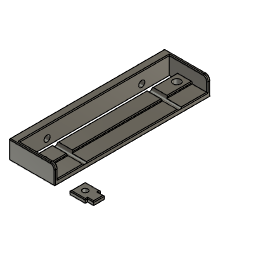
PS_LRS150-LM200_1515Mount (Autodesk Fusion 360 design; units mm, degrees)
Autodesk Fusion 360 part; units mm, degrees
sketch "Sketch1" plane through (0, 0, 0) normal (0, 0, 1) x (1, 0, 0)
  line L0 (0, 0) -> (5, 0)
  line L1 (5, 0) -> (5, 102)
  line L2 (5, 102) -> (0, 102)
  line L3 (0, 102) -> (0, 0)
  line L4 (5, 0) -> (5, 2)
  line L5 (5, 2) -> (5, 0)
  line L6 (5, 100) -> (5, 102)
  line L7 (0, 0) -> (30, 0)
  line L8 (30, 0) -> (30, 2)
  line L9 (30, 2) -> (0, 2)
  line L10 (0, 2) -> (0, 0)
  line L11 (0, 102) -> (30, 102)
  line L12 (30, 102) -> (30, 100)
  line L13 (30, 100) -> (0, 100)
  line L14 (0, 100) -> (0, 102)
  line L15 (0, 0) -> (30, 0)
  line L16 (30, 0) -> (30, 102)
  line L17 (30, 102) -> (0, 102)
  line L18 (0, 102) -> (0, 0)
  line L19 (5, 2) -> (10, 2)
  line L20 (10, 2) -> (20, 2)
  line L21 (20, 2) -> (20, 100)
  line L22 (20, 100) -> (10, 100)
  line L23 (10, 100) -> (10, 2)
  circle A0 centre (15, 7) radius 2.5
  circle A1 centre (15, 95) radius 2.5
  line L24 (40, 0) -> (54, 0)
  line L25 (54, 0) -> (54, 10)
  line L26 (54, 10) -> (40, 10)
  line L27 (40, 10) -> (40, 0)
  circle A2 centre (45, 5) radius 1.75
  line L28 (50, 0) -> (50, 1.5)
  line L29 (50, 1.5) -> (54, 1.5)
  line L30 (50, 10) -> (50, 8.5)
  line L31 (50, 8.5) -> (54, 8.5)
  point P0 (40, 0)
  dimension "d15" = 5
  dimension "d16" = 102
  dimension "d17" = 2
  dimension "d19" = 2
  dimension "d21" = 2
  dimension "d39" = 30
  dimension "d40" = 2
  dimension "d41" = 30
  dimension "d42" = 2
  dimension "d43" = 30
  dimension "d44" = 102
  dimension "d45" = 5
  dimension "d46" = 10
  dimension "d47" = 98
  dimension "d60" = 5
  dimension "d61" = 5
  dimension "d62" = 5
  dimension "d63" = 5
  dimension "d64" = 5
  dimension "d65" = 5
  dimension "d95" = 14
  dimension "d96" = 10
  dimension "d97" = 3.5
  dimension "d98" = 5
  dimension "d99" = 5
  dimension "d104" = 1.5
  dimension "d105" = 10
  dimension "d106" = 1.5
  constraint horizontal L0
  constraint vertical L1
  constraint horizontal L2
  constraint vertical L3
  constraint coincident L0.start L3.end
  constraint perpendicular L0 L4
  constraint horizontal L7
  constraint vertical L8
  constraint horizontal L9
  constraint vertical L10
  constraint horizontal L11
  constraint vertical L12
  constraint horizontal L13
  constraint vertical L14
  constraint horizontal L15
  constraint vertical L16
  constraint horizontal L17
  constraint vertical L18
  constraint perpendicular L5 L19
  constraint horizontal L20
  constraint vertical L21
  constraint horizontal L22
  constraint vertical L23
  constraint horizontal L24
  constraint vertical L25
  constraint horizontal L26
  constraint vertical L27
  constraint coincident P0 L24.start
  constraint coincident L24 L28.start
  constraint perpendicular L24 L28
  constraint coincident L25 L29.end
  constraint perpendicular L25 L29
  constraint coincident L26 L30.start
  constraint perpendicular L26 L30
  constraint coincident L25 L31.end
  constraint perpendicular L25 L31
  measures "d15" distance of L0.start L0.end
  measures "d16" distance of L0.start L2.end
  measures "d17" distance of L0.end L4.end
  measures "d19" distance of L0.end L4.end
  measures "d21" distance of L1.end L6.start
  measures "d39" distance of L0.start L7.end
  measures "d40" distance of L0.start L9.end
  measures "d41" distance of L2.end L11.end
  measures "d42" distance of L2.end L13.end
  measures "d43" distance of L0.start L7.end
  measures "d44" distance of L0.start L2.end
  measures "d45" distance of L4.end L19.end
  measures "d46" distance of L19.end L20.end
  measures "d47" distance of L19.end L22.end
  measures "d60" diameter of A0
  measures "d61" distance of L23 A0.centre
  measures "d62" distance of L9 A0.centre
  measures "d63" diameter of A1
  measures "d64" distance of L13 A1.centre
  measures "d65" distance of L23 A1.centre
  measures "d95" distance of P0 L24.end
  measures "d96" distance of P0 L26.end
  measures "d97" diameter of A2
  measures "d98" distance of L27 A2.centre
  measures "d99" distance of L24 A2.centre
  measures "d104" distance of L28.start L28.end
  measures "d105" distance of L27 L28
  measures "d106" distance of L30.start L30.end
extrude "Extrude1" add sketch "Sketch1" along normal blind 12 contours L0 L1 L3 L4 L5 L7 L9 L10 L15 L18 | L1 L4 L5 L7 L8 L9 L15 L16 L19 L20 | L1 L3 L9 L13 L18 | L1 L2 L3 L6 L11 L13 L14 L17 L18 | L1 L6 L11 L12 L13 L16 L17 L22 makes body 1
extrude "Extrude3" add sketch "Sketch1" along normal blind 4.25 contours L9 L13 L20 L21 L22 L23 | A0 | A1 bodies 1
fillet "Fillet3" radius 0.5 2 edges at (10, 51, 4.25) (20, 51, 4.25) on bodies 1
extrude "Extrude4" cut sketch "Sketch1" along normal blind 4.25 contours A0 | A1 bodies 1
sketch "Sketch2" plane through (0, 0, 0) normal (1, 0, 0) x (0, 1, 0)
  circle A0 centre (20, 4.5) radius 2
  circle A1 centre (82, 4.5) radius 2
  line L0 (0, 0) -> (0, 12.5)
  line L1 (102, 0) -> (102, 11)
  line L2 (102, 0) -> (0, 0)
  dimension "d68" = 4
  dimension "d69" = 4
  dimension "d70" = 20
  dimension "d73" = 4.5
  dimension "d74" = 4.5
  dimension "d75" = 20
  constraint coincident L0.start L2.end
  constraint vertical L0
  constraint vertical L1
  measures "d68" diameter of A0
  measures "d69" diameter of A1
  measures "d70" distance of A0.centre L0
  measures "d73" distance of A0.centre L2
  measures "d74" distance of A1.centre L2
  measures "d75" distance of A1.centre L1
extrude "Extrude5" add sketch "Sketch1" along normal blind 3 contours L9 L13 L16 L21 bodies 1
fillet "Fillet4" radius 3 2 edges at (30, 1, 12) (30, 101, 12) on bodies 1
fillet "Fillet5" radius 0.5 1 edges at (30, 51, 3) on bodies 1
fillet "Fillet6" radius 0.5 6 edges at (13.5, 0, 12) (29.1213, 0, 11.1213) (30, 0, 4.5) (30, 2, 5.75) (29.1213, 2, 11.1213) (16, 2, 12) on bodies 1
fillet "Fillet7" radius 0.5 7 edges at (5, 50.75, 12) (16, 100, 12) (29.1213, 100, 11.1213) (30, 100, 5.75) (30, 102, 4.5) (29.1213, 102, 11.1213) (13.5, 102, 12) on bodies 1
fillet "Fillet8" radius 0.5 5 edges at (0, 102, 5.75) (0, 101.8536, 11.8536) (0, 51, 12) (0, 0.1464, 11.8536) (0, 0, 5.75) on bodies 1
extrude "Extrude6" cut sketch "Sketch2" along normal blind 30 bodies 1
extrude "Extrude7" add sketch "Sketch1" along normal blind 2.5 separate body contours L24 L25 L26 L27 L28 L29 L30 L31 | L24 L25 L28 L29 | L25 L26 L30 L31 makes body 2
extrude "Extrude8" cut sketch "Sketch1" along normal blind 2.5 contours L24 L25 L28 L29 | L25 L26 L30 L31 bodies 2
chamfer "Chamfer1" distance 0.25 angle 45 8 edges at (52, 1.5, 0) (45, 0, 0) (50, 0.75, 0) (54, 5, 0) (52, 8.5, 0) (50, 9.25, 0) (45, 10, 0) (40, 5, 0) on bodies 2
chamfer "Chamfer2" distance 0.25 angle 45 8 edges at (30, 51, 0) (29.8536, 101.8536, 0) (15, 102, 0) (0.1464, 101.8536, 0) (0, 51, 0) (0.1464, 0.1464, 0) (15, 0, 0) (29.8536, 0.1464, 0) on bodies 1
fillet "Fillet13" radius 0.5 8 edges at (54, 5, 2.5) (52, 8.5, 2.5) (50, 9.25, 2.5) (45, 10, 2.5) (40, 5, 2.5) (45, 0, 2.5) (50, 0.75, 2.5) (52, 1.5, 2.5) on bodies 2
chamfer "Chamfer3" distance 0.25 angle 45 4 edges at (10, 51, 0) (7.5, 2, 0) (7.5, 100, 0) (5, 51, 0) on bodies 1
equation "SideWallThickness = 2 mm"
equation "BaseThickness = 3 mm"
equation "ClampBaseThickness = 1.25 mm"
equation "PowerSupplyWidth = 97 mm"
equation "ExtrusionMount = 5 mm"
equation "PS_MountLength = 30 mm"
equation "d15 = ExtrusionMount"
equation "d16 = SideWallThickness + PowerSupplyWidth + 1 mm + SideWallThickness"
equation "d17 = SideWallThickness"
equation "d19 = SideWallThickness"
equation "d21 = SideWallThickness"
equation "DistanceToPowerSupply = 20.5 mm"
equation "d39 = PS_MountLength"
equation "d40 = SideWallThickness"
equation "d41 = PS_MountLength"
equation "d42 = SideWallThickness"
equation "d43 = PS_MountLength"
equation "d44 = SideWallThickness + PowerSupplyWidth + 1 mm + SideWallThickness"
equation "d47 = PowerSupplyWidth + 1 mm"
named bodies: "PSMount_x2", "PSMountClamp_x4"
